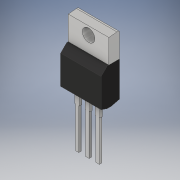
# Autodesk Inventor part: TO220
Saved by Autodesk Inventor 2017 (Build 210142000, 142)
## iProperties
Created: 2016-09-12
Part Number: TO220
Material: Rubber
Document SubType Name: Modeling
Designer: Home
Density: 0.93 g/cm^3
Appearance: Rubber - Black
Author: Home
Autodesk Inventor part; units mm, degrees
ref_plane "YZ Plane" through (0, 0, 0) normal (1, 0, 0) x (0, 1, 0)
ref_plane "XZ Plane" through (0, 0, 0) normal (0, 1, 0) x (-1, 0, 0)
ref_plane "XY Plane" through (0, 0, 0) normal (0, 0, 1) x (1, 0, 0)
sketch "Sketch1" plane through (0, 0, 0) normal (0, 1, 0) x (-1, 0, 0)
  line L0 (3.115, -0.3) -> (1.965, -0.3)
  line L1 (1.965, -0.3) -> (1.965, 0.3)
  line L2 (1.965, 0.3) -> (3.115, 0.3)
  line L3 (3.115, 0.3) -> (3.115, -0.3)
  line L4 (0.575, -0.3) -> (-0.575, -0.3)
  line L5 (-0.575, -0.3) -> (-0.575, 0.3)
  line L6 (-0.575, 0.3) -> (0.575, 0.3)
  line L7 (0.575, 0.3) -> (0.575, -0.3)
  line L8 (-1.965, -0.3) -> (-3.115, -0.3)
  line L9 (-3.115, -0.3) -> (-3.115, 0.3)
  line L10 (-3.115, 0.3) -> (-1.965, 0.3)
  line L11 (-1.965, 0.3) -> (-1.965, -0.3)
  point P0 (0, 0)
  point P1 (3.115, 0)
  point P2 (2.54, 0.3)
  point P3 (0, 0.3)
  point P4 (0.575, 0)
  point P5 (-2.54, 0.3)
  point P6 (-1.965, 0)
  point P7 (0, 0.3)
  dimension "d0" = 1.15
  dimension "d1" = 0.6
  dimension "d4" = 2.54
  constraints: 24 end point, 3 midpoint, 2 horizontal, 2 parallel, 1 collinear, 1 horizontal alignment, 1 perpendicular, 1 vertical alignment, 19 other
  measures "d0" distance of L0.start L0.end
  measures "d1" distance of L0.end L1.end
  measures "d4" distance of L0.start L4.start
extrude "Extrusion1" add sketch "Sketch1" along normal blind 3
sketch "Sketch2" plane through (0, 0, 0) normal (0, -1, 0) x (1, 0, 0)
  line L0 (-0.575, 0.3) -> (0.575, 0.3) projected
  line L1 (0.575, -0.3) -> (-0.575, -0.3) projected
  line L2 (-0.425, 0.3) -> (0.425, 0.3)
  line L3 (0.425, 0.3) -> (0.425, -0.3)
  line L4 (0.425, -0.3) -> (-0.425, -0.3)
  line L5 (-0.425, -0.3) -> (-0.425, 0.3)
  line L6 (-3.115, 0.3) -> (-1.965, 0.3) projected
  line L7 (-2.965, 0.3) -> (-2.115, 0.3)
  line L8 (-2.115, 0.3) -> (-2.115, -0.3)
  line L9 (-2.115, -0.3) -> (-2.965, -0.3)
  line L10 (-2.965, -0.3) -> (-2.965, 0.3)
  line L11 (1.965, 0.3) -> (3.115, 0.3) projected
  line L12 (3.115, -0.3) -> (1.965, -0.3) projected
  line L13 (2.115, 0.3) -> (2.965, 0.3)
  line L14 (2.965, 0.3) -> (2.965, -0.3)
  line L15 (2.965, -0.3) -> (2.115, -0.3)
  line L16 (2.115, -0.3) -> (2.115, 0.3)
  line L17 (-1.965, -0.3) -> (-3.115, -0.3) projected
  point P0 (0, 0)
  point P1 (-2.54, 0.3)
  point P2 (-2.54, -0.3)
  point P3 (0, -0.3)
  point P4 (2.54, -0.3)
  dimension "d11" = 0.85
  dimension "d12" = 0.85
  dimension "d13" = 0.85
  dimension "d14" = 2.54
  constraints: 24 end point, 6 parallel, 6 point on line, 4 midpoint, 3 horizontal, 3 perpendicular, 2 vertical alignment
  measures "d11" distance of L8.end L9.end
  measures "d12" distance between parallel lines of L3 L5
  measures "d13" distance between parallel lines of L14 L16
  measures "d14" horizontal distance of point (0, 0) point (2.54, -0.3)
extrude "Extrusion2" add sketch "Sketch2" along normal blind 10
sketch "Sketch3" plane through (0, 3, 0) normal (0, 1, 0) x (1, 0, 0)
  line L0 (5, 2.6) -> (-5, 2.6)
  line L1 (-5, 2.6) -> (-5, -1.9)
  line L2 (-5, -1.9) -> (5, -1.9)
  line L3 (5, -1.9) -> (5, 2.6)
  point P0 (0, 0)
  point P1 (0, -1.9)
  dimension "d17" = 4.5
  dimension "d18" = 2.6
  dimension "d19" = 10
  constraints: 8 end point, 2 parallel, 1 horizontal, 1 midpoint, 1 perpendicular, 1 vertical alignment
  measures "d17" distance of L0.end L1.end
  measures "d18" distance from line of point (0, 0) L0
  measures "d19" distance of L1.end L2.end
extrude "Extrusion3" add sketch "Sketch3" along normal blind 9.1 separate body
sketch "Sketch4" plane through (0, 12.1, 0) normal (0, 1, 0) x (1, 0, 0)
  line L0 (5, 2.6) -> (-5, 2.6) projected
  line L1 (-5, 2.6) -> (-5, -1.9) projected
  line L2 (5, 2.6) -> (-5, 2.6)
  line L3 (-5, 2.6) -> (-5, 0)
  line L4 (-5, 0) -> (5, 0)
  line L5 (5, 0) -> (5, 2.6)
  point P0 (0, 0)
  dimension "d22" = 2.6
  constraints: 8 end point, 2 parallel, 1 horizontal, 1 perpendicular, 1 point on line
  measures "d22" distance between parallel lines of L4 L0
extrude "Extrusion4" add sketch "Sketch4" along normal blind 6.1 bodies 1
sketch "Sketch5" plane through (-5, 12.1, 0) normal (0, 0, 1) x (1, 0, 0)
  circle A0 centre (5, 3.9) radius 1.55
  line L0 (0, -9.1) -> (10, -9.1) projected
  point P0 (5, -12.1)
  point P1 (5.425, -12.1)
  dimension "d25" = 16
  dimension "d26" = 3.1
  constraints: 1 centre point
  measures "d25" vertical distance of point (5.425, -12.1) A0.centre
  measures "d26" diameter of A0
extrude "Extrusion5" cut sketch "Sketch5" against normal through all bodies 1
chamfer "Chamfer1" distance 0.5 distance2 2 1 edges at (0, 3, -2.6) measured on face at (1.6667, 6.0333, -2.6)
chamfer "Chamfer2" distance 0.5 distance2 1.5 1 edges at (0, 3, 1.9) measured on face at (-1.6667, 6.0333, 1.9)
chamfer "Chamfer3" distance 1.5 distance2 1.5 1 edges at (0, 12.1, 1.9) measured on face at (-1.6667, 12.1, -1.1)
chamfer "Chamfer4" distance 2 distance2 0.2 1 edges at (0, 18.2, 0) measured on face at (-1.6667, 18.2, -0.8667)
chamfer "Chamfer5" distance 0.2 distance2 0.2 1 edges at (0, 18.2, -2.6) measured on face at (-1.6667, 18.2, -2.2)
equation "\"d0\" = fF1"
equation "\"d1\" = fE"
equation "\"d9\" = fG"
equation "\"d11\" = fF2"
equation "\"d12\" = fF2"
equation "\"d13\" = fF2"
equation "\"d15\" = fL4"
equation "\"d17\" = fA1"
equation "\"d18\" = fD1"
equation "\"d20\" = fL7"
equation "\"d22\" = fB1"
equation "\"d23\" = fL6 - fL7"
equation "\"d25\" = fL2"
equation "\"d26\" = fDia"
equation "\"d27\" = fL6 - fL7"
equation "\"fE\" = 0.6"
equation "\"fF1\" = 1.15"
equation "\"fG\" = 3"
equation "\"fF2\" = 0.85"
equation "\"fL4\" = 10"
equation "\"fA1\" = 4.5"
equation "\"fD1\" = 2.6"
equation "\"fH1\" = 1"
equation "\"fL7\" = 9.1"
equation "\"fB1\" = 2.6"
equation "\"fL6\" = 15.2"
equation "\"fL2\" = 16"
equation "\"fDia\" = 3.1"
body "Solid1"
body "Solid2"
